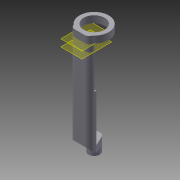
# Autodesk Inventor part: MU_Motor_Asm_Frame_new3
Saved by Autodesk Inventor 2011 SP2 (Build 150309200, 309)
## iProperties
Created: 2011-09-08
Part Number: MU_Motor_Asm_Frame_new3
Document SubType Name: Modeling
Designer: sungwook
Density: 2.71 g/cm^3
Material: Aluminum-6061
Author: sungwook
Autodesk Inventor part; units mm, degrees
ref_plane "YZ Plane" through (0, 0, 0) normal (1, 0, 0) x (0, 1, 0)
ref_plane "XZ Plane" through (0, 0, 0) normal (0, 1, 0) x (-1, 0, 0)
ref_plane "XY Plane" through (0, 0, 0) normal (0, 0, 1) x (1, 0, 0)
sketch "Sketch1" plane through (0, 0, 0) normal (0, 0, 1) x (1, 0, 0)
  line L0 (-1.39, -1.09) -> (1.39, -1.09)
  line L1 (1.39, -1.09) -> (1.39, -2.09)
  line L2 (1.39, -2.09) -> (-1.39, -2.09)
  line L3 (-1.39, -2.09) -> (-1.39, -1.09)
  point P0 (0, 0)
  dimension "d0" = 1
  dimension "d1" = 1.39
  dimension "d2" = 2.78
  dimension "d3" = 1.09
  constraints: 8 end point, 2 parallel, 1 horizontal, 1 perpendicular
  measures "d0" distance of L2.end L0.start
  measures "d1" distance from line of L1 point (0, 0)
  measures "d2" distance of L1.end L2.end
  measures "d3" distance from line of L0 point (0, 0)
extrude "Extrusion1" add sketch "Sketch1" along normal blind 15.9
sketch "Sketch2" plane through (-1.39, -1.09, 0) normal (0, 1, 0) x (1, 0, 0)
  line L0 (0, 0) -> (0, -15.9) projected
  line L1 (0, -8.8) -> (2.78, -8.8)
  line L2 (2.78, -8.8) -> (2.78, -15.9)
  line L3 (2.78, -15.9) -> (0, -15.9)
  line L4 (0, -15.9) -> (0, -8.8)
  point P0 (1.39, 0)
  dimension "d6" = 7.1
  constraints: 8 end point, 2 parallel, 1 horizontal, 1 perpendicular, 1 point on line
  measures "d6" distance of L3.end L1.start
extrude "Extrusion2" cut sketch "Sketch2" against normal blind 0.2685
sketch "Sketch3" plane through (0, 0, 0) normal (0, 0, -1) x (-1, 0, 0)
  line L0 (-1.39, -1.09) -> (1.39, -1.09)
  line L1 (1.39, -1.09) -> (1.39, 1.69)
  line L2 (1.39, 1.69) -> (-1.39, 1.69)
  line L3 (-1.39, 1.69) -> (-1.39, -1.09)
  point P0 (0, 0)
  dimension "d9" = 2.78
  constraints: 8 end point, 2 parallel, 1 horizontal, 1 perpendicular
  measures "d9" distance of L2.end L0.start
extrude "Extrusion3" add sketch "Sketch3" against normal blind 2
sketch "Sketch4" plane through (0, 0, 0) normal (0, 0, -1) x (-1, 0, 0)
  line L0 (-1.39, 1.69) -> (-1.39, -2.09) projected
  line L1 (1.39, -2.09) -> (1.39, 1.69) projected
  line L2 (1.39, 1.69) -> (-1.39, 1.69) projected
  circle A0 centre (0, 0) radius 0.8
  line L3 (-1.39, -1.3585) -> (1.39, -1.3585) projected
  line L4 (-1.39, -1.09) -> (1.39, -1.09) projected
  line L5 (-1.39, -1.09) -> (-0.7252, 0.3377)
  line L6 (1.39, -1.09) -> (0.7252, 0.3377)
  dimension "d12" = 1.6
  constraints: 4 end point, 2 point on circle, 2 tangent, 1 centre point, 1 coincident
  measures "d12" diameter of A0
extrude "Extrusion4" cut sketch "Sketch4" against normal through all contours L2 L1 L6 A0 L5 L0
sketch "Sketch5" plane through (0, 0, 0) normal (0, 0, -1) x (-1, 0, 0)
  line L0 (-0.7252, 0.3377) -> (-1.39, -1.09) projected
  line L1 (-1.39, -1.09) -> (-1.39, -2.09) projected
  line L2 (-1.39, -2.09) -> (1.39, -2.09) projected
  line L3 (1.39, -2.09) -> (1.39, -1.09) projected
  line L4 (1.39, -1.09) -> (0.7252, 0.3377) projected
  arc A0 (0.7252, 0.3377) -> (-0.7252, 0.3377) centre (0, 0) ccw projected
  circle A1 centre (0, 0) radius 0.8
  constraints: 1 centre point, 1 coincident, 1 tangent
extrude "Extrusion5" cut sketch "Sketch5" against normal blind 1 contours A1 L4 L3 L2 L1 L0
hole "Hole1" at (0, 0, 0) direction (0, 0, 1) diameter 0.5 depth 1.7 countersink diameter 1 countersink angle 90
sketch "Sketch6" plane through (-1.39, -2.09, 15.9) normal (0, -1, 0) x (1, 0, 0)
  line L0 (2.78, -15.9) -> (2.78, 0) projected
  line L1 (2.78, 0) -> (0, 0) projected
  circle A0 centre (1.39, -1.5) radius 0.5
  point P0 (2.78, -14.9)
  point P1 (1.39, -15.9)
  point P2 (1.39, -1)
  point P3 (1.39, -2)
  dimension "d26" = 1
  dimension "d27" = 1.39
  dimension "d28" = 1.5
  constraints: 2 point on circle, 1 centre point
  measures "d26" diameter of A0
  measures "d27" distance from line of L0 A0.centre
  measures "d28" distance from line of A0.centre L1
extrude "Extrusion6" [suppressed]
chamfer "Chamfer1" distance 1 angle 45 1 edges at (0, -2.09, 1)
ref_plane "Work Plane1" through (0, -2.09, 14.9) normal (0, 0, 1) x (1, 0, 0)
ref_plane "Work Plane2" through (0, -2.09, 13.9) normal (0, 0, 1) x (1, 0, 0)
sketch "Sketch10" plane through (0, 0, 15.9) normal (0, 0, 1) x (1, 0, 0)
  line L0 (1.39, -1.3585) -> (-1.39, -1.3585) projected
  circle A0 centre (0, 0) radius 2.09
  line L1 (1.39, -2.09) -> (-1.39, -2.09) projected
  dimension "d54" = 4.18
  constraints: 1 centre point, 1 coincident, 1 tangent
  measures "d54" diameter of A0
extrude "Extrusion7" add sketch "Sketch10" against normal blind 1
sketch "Sketch11" plane through (0, 0, 15.9) normal (0, 0, 1) x (1, 0, 0)
  arc A0 (1.39, -1.5608) -> (-1.39, -1.5608) centre (0, 0) ccw projected
  circle A1 centre (0, 0) radius 1.3
  point P0 (1.6431, -0.954)
  point P1 (-1.6431, -0.954)
  dimension "d41" = 2.6
  constraints: 1 centre point, 1 coincident, 1 other
  measures "d41" diameter of A1
hole "Hole2" at (0, 0, 15.9) direction (0, 0, -1) diameter 3 depth 1.1
fillet "Fillet3" radius 0.7 2 edges at (1.39, -2.09, 8.95) (-1.39, -2.09, 8.95)
sketch "Sketch13" plane through (-1.39, -1.09, 8.8) normal (0, 0, 1) x (1, 0, 0)
  point P0 (1.39, 1.09)
  point P1 (1.39, 1.09)
  constraints: 1 coincident
hole "Hole4" at (0, 0, 8.8) at (0, 0, 8.8) direction (0, 0, -1) diameter 2.8 depth 6.8
sketch "Sketch15" plane through (0, -2.09, 14.9) normal (0, 0, 1) x (1, 0, 0)
  point P0 (0, 2.09)
  point P1 (0, 2.09)
  constraints: 1 coincident
hole "Hole5" [suppressed]
body "Solid1"
